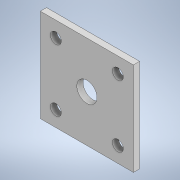
# Autodesk Inventor part: 3SR15_ポテンショメータ固定パーツ
Saved by Autodesk Inventor 2021 (Build 250183000, 183)
## iProperties
Created: 2021-04-24
Part Number: 3SR15_ポテンショメータ固定パーツ
Material: 一般
Document SubType Name: Modeling
Designer: ryusei
Density: 1 g/cm^3
Appearance: 既定
Author: ryusei
Autodesk Inventor part; units mm, degrees
ref_plane "YZ Plane" through (0, 0, 0) normal (1, 0, 0) x (0, 1, 0)
ref_plane "XZ Plane" through (0, 0, 0) normal (0, 1, 0) x (-1, 0, 0)
ref_plane "XY Plane" through (0, 0, 0) normal (0, 0, 1) x (1, 0, 0)
sketch "スケッチ1" plane through (0, 0, 0) normal (0, 0, 1) x (1, 0, 0)
  line L0 (0, 0) -> (30, 0)
  line L1 (30, 0) -> (30, 30)
  line L2 (30, 30) -> (0, 30)
  line L3 (0, 30) -> (0, 0)
  dimension "d0" = 30
  dimension "d1" = 30
  constraints: 8 end point, 2 parallel, 1 horizontal, 1 perpendicular
  measures "d0" distance between parallel lines of L1 L3
  measures "d1" distance between parallel lines of L0 L2
extrude "押し出し1" add sketch "スケッチ1" along normal blind 2
sketch "スケッチ2" plane through (0, 0, 2) normal (0, 0, 1) x (1, 0, 0)
  line L0 (30, 0) -> (30, 30) projected
  line L1 (30, 30) -> (0, 30) projected
  line L2 (0, 30) -> (0, 0) projected
  line L3 (0, 0) -> (30, 0) projected
  point P0 (25, 25)
  point P1 (5, 25)
  point P2 (5, 5)
  point P3 (25, 5)
  dimension "d4" = 5
  dimension "d5" = 5
  dimension "d6" = 5
  dimension "d7" = 5
  dimension "d8" = 5
  dimension "d9" = 5
  dimension "d10" = 5
  dimension "d11" = 5
  measures "d4" distance from line of L0 point (25, 25)
  measures "d5" distance from line of L1 point (25, 25)
  measures "d6" distance from line of L1 point (5, 25)
  measures "d7" distance from line of point (5, 25) L2
  measures "d8" distance from line of L3 point (5, 5)
  measures "d9" distance from line of L2 point (5, 5)
  measures "d10" distance from line of L3 point (25, 5)
  measures "d11" distance from line of L0 point (25, 5)
hole "穴1" at (25, 25, 2) at (5, 25, 2) at (5, 5, 2) at (25, 5, 2) direction (0, 0, -1) diameter 3.5 end through all
sketch "スケッチ3" plane through (0, 0, 2) normal (0, 0, 1) x (1, 0, 0)
  line L0 (30, 0) -> (30, 30) projected
  line L1 (30, 30) -> (0, 30) projected
  point P0 (0, 0)
  point P1 (15, 15)
  dimension "d19" = 15
  dimension "d20" = 15
  measures "d19" distance from line of L0 point (15, 15)
  measures "d20" distance from line of L1 point (15, 15)
hole "穴2" at (15, 15, 2) direction (0, 0, -1) diameter 6.5 end through all
